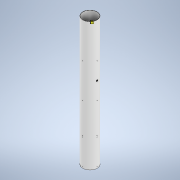
# Autodesk Inventor part: Tubo Central
Saved by Autodesk Inventor 2020 (Build 240168000, 168)
## iProperties
Created: 2021-10-16
Part Number: Tubo Central
Material: PVC-Piping
Document SubType Name: Modeling
Designer: Carlos
Density: 1.4 g/cm^3
Appearance: Smooth - White
Mass: 273.965 g
Surface Area: 2950.7 cm^2
Volume: 195.689 cm^3
Author: Carlos
Autodesk Inventor part; units mm, degrees
ref_plane "YZ Plane" through (0, 0, 0) normal (1, 0, 0) x (0, 1, 0)
ref_plane "XZ Plane" through (0, 0, 0) normal (0, 1, 0) x (-1, 0, 0)
ref_plane "XY Plane" through (0, 0, 0) normal (0, 0, 1) x (1, 0, 0)
sketch "Sketch1" plane through (0, 0, 0) normal (0, 1, 0) x (-1, 0, 0)
  circle A0 centre (0, 0) radius 36.5
  circle A1 centre (0, 0) radius 35.17
  dimension "d0" = 73
  dimension "d89" = 1.33
  dimension "d90" = 70.34
  constraints: 2 centre point, 2 coincident
  measures "d0" diameter of A0
  measures "d89" radial gap between concentric circles of A0 A1
  measures "d90" diameter of A1
extrude "Extrusion1" add sketch "Sketch1" along normal mid plane 654
sketch "Sketch2" plane through (0, 0, 0) normal (1, 0, 0) x (0, 1, 0)
  line L0 (327, -36.5) -> (327, 36.5) projected
  line L1 (327, 36.5) -> (147, 36.5)
  line L2 (-327, 36.5) -> (327, 36.5) projected
  line L3 (147, 36.5) -> (147, -36.5)
  line L4 (-327, -36.5) -> (327, -36.5) projected
  point P0 (0, 0)
  point P1 (147, 0)
  dimension "d4" = 180
  constraints: 4 end point, 2 point on line, 1 midpoint, 1 perpendicular
  measures "d4" distance of L0.end L1.end
hole "Hole1" at (0, 147, 0) direction (-1, 0, 0) diameter 2 depth 76 tip angle 118
pattern_circular "Circular Pattern1" count 4 over 360 about axis through (0, -10, 0) along (0, 1, 0) of "Hole1"
thread "Thread1" size "M2x0.4" class "6H" standard "ANSI Metric M Profile" full length
thread "Thread2" size "M2x0.4" class "6H" standard "ANSI Metric M Profile" full length
thread "Thread3" size "M2x0.4" class "6H" standard "ANSI Metric M Profile" full length
thread "Thread4" size "M2x0.4" class "6H" standard "ANSI Metric M Profile" full length
sketch "Sketch3" plane through (0, 0, 0) normal (0, 0, 1) x (1, 0, 0)
  line L0 (36.5, 327) -> (-36.5, 327) projected
  line L1 (36.5, 327) -> (36.5, -28)
  line L2 (36.5, -327) -> (36.5, 327) projected
  line L3 (36.5, -28) -> (-36.5, -28)
  line L4 (-36.5, -327) -> (-36.5, 327) projected
  point P0 (0, 0)
  point P1 (0, -28)
  point P2 (0, -28)
  dimension "d23" = 355
  constraints: 4 end point, 2 point on line, 1 coincident, 1 horizontal, 1 midpoint
  measures "d23" distance of L0.start L1.end
hole "Hole2" at (0, -28, 0) direction (0, 0, -1) diameter 2 depth 76 tip angle 118
thread "Thread9" size "M2x0.4" class "6H" standard "ANSI Metric M Profile" full length
pattern_circular "Circular Pattern2" count 4 over 360 about axis through (0, -10, 0) along (0, 1, 0) of "Hole2"
sketch "Sketch4" plane through (0, 0, 0) normal (1, 0, 0) x (0, 1, 0)
  line L0 (-327, -35.17) -> (-327, 35.17) projected
  line L1 (-327, 35.17) -> (-182.5, 35.17)
  line L2 (327, 35.17) -> (-327, 35.17) projected
  line L3 (-182.5, 35.17) -> (-182.5, -36.5)
  line L4 (-327, -36.5) -> (327, -36.5) projected
  point P0 (0, 0)
  point P1 (-182.5, -0.665)
  dimension "d36" = 144.5
  constraints: 4 end point, 2 point on line, 1 midpoint, 1 perpendicular
  measures "d36" distance of L0.end L1.end
hole "Hole3" at (0, -182.5, -0.665) direction (-1, 0, 0) diameter 2 depth 76 tip angle 118
pattern_circular "Circular Pattern3" count 4 over 360 about axis through (0, -10, 0) along (0, 1, 0) of "Hole3"
sketch "Sketch6" plane through (0, 0, 0) normal (0, 0, 1) x (1, 0, 0)
  line L0 (-36.5, -327) -> (36.5, -327) projected
  line L1 (-36.5, -327) -> (-35.17, -189.0064)
  line L2 (-35.17, 327) -> (-35.17, -327) projected
  line L3 (-35.17, -189.0064) -> (36.5, -189.0064)
  line L4 (36.5, -327) -> (36.5, 327) projected
  point P0 (0, 0)
  point P1 (0.665, -189.0064)
  dimension "d50" = 138
  constraints: 4 end point, 2 point on line, 1 horizontal, 1 midpoint
  measures "d50" distance of L0.start L1.end
hole "Hole4" at (0.665, -189.0064, 0) direction (0, 0, -1) diameter 2 depth 76 tip angle 118
pattern_circular "Circular Pattern4" count 4 over 360 about axis through (0, -10, 0) along (0, 1, 0) of "Hole4"
sketch "Sketch7" plane through (0, 0, 0) normal (1, 0, 0) x (0, 1, 0)
  line L0 (-327, 36.5) -> (327, 36.5) projected
  line L1 (327, -35.17) -> (-327, -35.17) projected
  line L2 (-327, 36.5) -> (-318, 36.5)
  line L3 (-327, 36.5) -> (327, 36.5) projected
  line L4 (-318, 36.5) -> (-318, 0)
  point P0 (0, 0)
  dimension "d87" = 9
  constraints: 4 end point, 1 coincident, 1 perpendicular, 1 point on line
  measures "d87" distance of L0.start L2.end
hole "Hole5" at (0, -318, 0) direction (1, 0, 0) diameter 2 depth 76 tip angle 118
pattern_circular "Circular Pattern5" count 4 over 360 about axis through (0, -10, 0) along (0, 1, 0) of "Hole5"
sketch "Sketch8" plane through (0, 0, 0) normal (1, 0, 0) x (0, 1, 0)
  line L0 (-327, 36.5) -> (327, 36.5) projected
  line L1 (432, 36.5) -> (72, 36.5)
  circle A0 centre (147, 0) radius 0.9998
  line L2 (147, 0) -> (-28, 0)
  point P0 (0, 0)
  point P1 (147, -1)
  point P2 (0, 0)
  point P3 (147, 1)
  point P4 (59.5, 0)
  constraints: 4 end point, 2 point on line, 2 vertical alignment, 1 centre point, 1 coincident, 1 midpoint
hole "Hole6" at (0, 59.5, 0) direction (1, 0, 0) diameter 8.382 depth 76 tip angle 118
thread "Thread10" size "M2x0.4" class "6H" standard "ANSI Metric M Profile" full length
thread "Thread11" size "M2x0.4" class "6H" standard "ANSI Metric M Profile" full length
thread "Thread12" size "M2x0.4" class "6H" standard "ANSI Metric M Profile" full length
thread "Thread13" size "M2x0.4" class "6H" standard "ANSI Metric M Profile" full length
thread "Thread14" size "M2x0.4" class "6H" standard "ANSI Metric M Profile" full length
thread "Thread15" size "M2x0.4" class "6H" standard "ANSI Metric M Profile" full length
thread "Thread16" size "M2x0.4" class "6H" standard "ANSI Metric M Profile" full length
thread "Thread17" size "M2x0.4" class "6H" standard "ANSI Metric M Profile" full length
thread "Thread18" size "M2x0.4" class "6H" standard "ANSI Metric M Profile" full length
thread "Thread19" size "M2x0.4" class "6H" standard "ANSI Metric M Profile" full length
thread "Thread20" size "M2x0.4" class "6H" standard "ANSI Metric M Profile" full length
thread "Thread21" size "M2x0.4" class "6H" standard "ANSI Metric M Profile" full length
thread "Thread22" size "M2x0.4" class "6H" standard "ANSI Metric M Profile" full length
thread "Thread23" size "M2x0.4" class "6H" standard "ANSI Metric M Profile" full length
thread "Thread24" size "M2x0.4" class "6H" standard "ANSI Metric M Profile" full length
body "Solid1"
